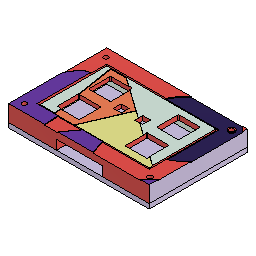
hackpaddelta (Autodesk Fusion 360 design; units mm, degrees)
part number: 2026-03-17-23-30-56-506
Autodesk Fusion 360 part; units mm, degrees
sketch "Sketch3" plane through (0, 0, 0) normal (0, 0, 1) x (1, 0, 0)
  line L0 (0, 0) -> (69.5, 0)
  line L1 (69.5, 0) -> (69.5, 42.5)
  line L2 (69.5, 42.5) -> (0, 42.5)
  line L3 (0, 42.5) -> (0, 0)
  dimension "d5" = 69.5
  dimension "d6" = 42.5
  constraint horizontal L0
  constraint vertical L1
  constraint horizontal L2
  constraint vertical L3
  constraint coincident L0.start L3.end
  measures "d5" distance of L0.start L0.end
  measures "d6" distance of L0.start L2.end
sketch "Sketch11" plane through (0, 0, 0) normal (0, 0, 1) x (1, 0, 0)
  line L0 (0, 0) -> (69.5, 0)
  line L1 (69.5, 0) -> (69.5, 42.5)
  line L2 (69.5, 42.5) -> (0, 42.5)
  line L3 (0, 42.5) -> (0, 0)
  dimension "d46" = 69.5
  dimension "d47" = 42.5
  constraint horizontal L0
  constraint vertical L1
  constraint horizontal L2
  constraint vertical L3
  measures "d46" distance of L0.start L0.end
  measures "d47" distance of L0.start L2.end
sketch "Sketch5" plane through (0, 0, 0) normal (0, 0, 1) x (1, 0, 0)
  line L0 (0, 0) -> (69.5, 0)
  line L1 (69.5, 0) -> (69.5, 42.5)
  line L2 (69.5, 42.5) -> (0, 42.5)
  line L3 (0, 42.5) -> (0, 0)
  line L4 (-10, -10) -> (79.5, -10)
  line L5 (79.5, -10) -> (79.5, 52.5)
  line L6 (79.5, 52.5) -> (-10, 52.5)
  line L7 (-10, 52.5) -> (-10, -10)
  circle A0 centre (-5, 47) radius 1.45
  circle A1 centre (-5, -5) radius 1.45
  circle A2 centre (75, 47) radius 1.45
  circle A3 centre (75, -5) radius 1.45
  dimension "d9" = 69.5
  dimension "d10" = 42.5
  dimension "d11" = 10
  dimension "d12" = 2.9
  dimension "d13" = 2.9
  dimension "d14" = 2.9
  dimension "d15" = 2.9
  constraint horizontal L0
  constraint vertical L1
  constraint horizontal L2
  constraint vertical L3
  constraint coincident L0.start L3.end
  measures "d9" distance of L0.start L0.end
  measures "d10" distance of L0.start L2.end
  measures "d12" diameter of A0
  measures "d13" diameter of A1
  measures "d14" diameter of A2
  measures "d15" diameter of A3
extrude "Extrude1" add sketch "Sketch5" along normal blind 3 contours L0 L1 L2 L3 makes body 1
extrude "Extrude2" add sketch "Sketch5" along normal blind 3 separate body makes body 2
sketch "Sketch6" plane through (0, 0, 3) normal (0, 0, 1) x (-1, 0, 0)
  line L0 (-25.0112, -26.63) -> (-30.0112, -26.63)
  line L1 (-30.0112, -26.63) -> (-30.0112, -21.63)
  line L2 (-30.0112, -21.63) -> (-25.0112, -21.63)
  line L3 (-25.0112, -21.63) -> (-25.0112, -26.63)
  line L4 (-43.6881, -26.63) -> (-38.6881, -26.63)
  line L5 (-38.6881, -26.63) -> (-38.6881, -21.63)
  line L6 (-38.6881, -21.63) -> (-43.6881, -21.63)
  line L7 (-43.6881, -21.63) -> (-43.6881, -26.63)
  dimension "d36" = 5
  dimension "d37" = 5
  dimension "d40" = 5
  dimension "d41" = 5
  constraint horizontal L0
  constraint vertical L1
  constraint horizontal L2
  constraint vertical L3
  constraint horizontal L4
  constraint vertical L5
  constraint horizontal L6
  constraint vertical L7
  measures "d36" distance of L0.start L0.end
  measures "d37" distance of L0.start L2.end
  measures "d40" distance of L4.start L4.end
  measures "d41" distance of L4.start L6.end
extrude "Extrude3" add 1 faces at (73.5198, 14, 3) along direction (0, 0, 1) blind 10 separate body on bodies 2 makes body 3
sketch "Sketch7" plane through (0, 0, 3) normal (0, 0, 1) x (-1, 0, 0)
  arc A0 (-20.375, -18.025) -> (-19.875, -18.525) centre (-19.875, -18.025) ccw
  arc A1 (-6.875, -18.525) -> (-6.375, -18.025) centre (-6.875, -18.025) ccw
  arc A2 (-6.375, -5.025) -> (-6.875, -4.525) centre (-6.875, -5.025) ccw
  arc A3 (-19.875, -4.525) -> (-20.375, -5.025) centre (-19.875, -5.025) ccw
  line L0 (-19.875, -18.525) -> (-6.875, -18.525)
  line L1 (-6.875, -4.525) -> (-19.875, -4.525)
  line L2 (-6.375, -18.025) -> (-6.375, -5.025)
  line L3 (-20.375, -5.025) -> (-20.375, -18.025)
  arc A4 (-6.375, -25.025) -> (-6.875, -24.525) centre (-6.875, -25.025) ccw
  line L4 (-19.875, -38.525) -> (-6.875, -38.525)
  arc A5 (-6.875, -38.525) -> (-6.375, -38.025) centre (-6.875, -38.025) ccw
  arc A6 (-20.375, -38.025) -> (-19.875, -38.525) centre (-19.875, -38.025) ccw
  line L5 (-6.875, -24.525) -> (-19.875, -24.525)
  line L6 (-20.375, -25.025) -> (-20.375, -38.025)
  arc A7 (-19.875, -24.525) -> (-20.375, -25.025) centre (-19.875, -25.025) ccw
  line L7 (-6.375, -38.025) -> (-6.375, -25.025)
  arc A8 (-50.125, -18.525) -> (-49.625, -18.025) centre (-50.125, -18.025) ccw
  line L8 (-50.125, -4.525) -> (-63.125, -4.525)
  arc A9 (-63.125, -4.525) -> (-63.625, -5.025) centre (-63.125, -5.025) ccw
  arc A10 (-49.625, -5.025) -> (-50.125, -4.525) centre (-50.125, -5.025) ccw
  line L9 (-63.625, -5.025) -> (-63.625, -18.025)
  line L10 (-49.625, -18.025) -> (-49.625, -5.025)
  line L11 (-63.125, -18.525) -> (-50.125, -18.525)
  arc A11 (-63.625, -18.025) -> (-63.125, -18.525) centre (-63.125, -18.025) ccw
  arc A12 (-63.625, -38.025) -> (-63.125, -38.525) centre (-63.125, -38.025) ccw
  arc A13 (-63.125, -24.525) -> (-63.625, -25.025) centre (-63.125, -25.025) ccw
  line L12 (-63.625, -25.025) -> (-63.625, -38.025)
  line L13 (-50.125, -24.525) -> (-63.125, -24.525)
  line L14 (-49.625, -38.025) -> (-49.625, -25.025)
  line L15 (-63.125, -38.525) -> (-50.125, -38.525)
  arc A14 (-50.125, -38.525) -> (-49.625, -38.025) centre (-50.125, -38.025) ccw
  arc A15 (-49.625, -25.025) -> (-50.125, -24.525) centre (-50.125, -25.025) ccw
extrude "Extrude4" add 1 faces at (23.1667, 14.1667, 3) along direction (0, 0, -1) blind 3 from surface at -10 on bodies 1 bodies 1 3
extrude "Extrude5" cut sketch "Sketch7" sketch "Sketch6" against normal blind 10 from surface at 10 of sketch 2 bodies 3
sketch "Sketch13" plane through (0, -10, 0) normal (0, -1, 0) x (1, 0, 0)
  line L0 (-10, 3) -> (79.5, 3)
  line L1 (79.5, 3) -> (79.5, 13)
  line L2 (79.5, 13) -> (-10, 13)
  line L3 (-10, 13) -> (-10, 3)
  line L4 (20.5, 9) -> (49.5, 9)
  line L5 (49.5, 9) -> (49.5, 3)
  line L6 (49.5, 3) -> (20.5, 3)
  line L7 (20.5, 3) -> (20.5, 9)
  dimension "d54" = 6
  constraint horizontal L4
  constraint vertical L5
  constraint horizontal L6
  constraint vertical L7
  measures "d54" distance of L4.start L6.end
extrude "Extrude6" cut sketch "Sketch13" against normal blind 10 contours L0 L4 L5 L6 L7 bodies 3
sketch "Sketch14" plane through (0, 0, 13) normal (0, 0, 1) x (-1, 0, 0)
  line L0 (-38.6881, -26.63) -> (-43.6881, -26.63)
  line L1 (-43.6881, -26.63) -> (-43.6881, -21.63)
  line L2 (-43.6881, -21.63) -> (-38.6881, -21.63)
  line L3 (-38.6881, -21.63) -> (-38.6881, -26.63)
  arc A0 (-20.375, -18.025) -> (-19.875, -18.525) centre (-19.875, -18.025) ccw
  line L4 (-20.375, -18.025) -> (-20.375, -5.025)
  arc A1 (-19.875, -4.525) -> (-20.375, -5.025) centre (-19.875, -5.025) ccw
  line L5 (-19.875, -4.525) -> (-6.875, -4.525)
  arc A2 (-6.375, -5.025) -> (-6.875, -4.525) centre (-6.875, -5.025) ccw
  line L6 (-6.375, -5.025) -> (-6.375, -18.025)
  arc A3 (-6.875, -18.525) -> (-6.375, -18.025) centre (-6.875, -18.025) ccw
  line L7 (-6.875, -18.525) -> (-19.875, -18.525)
  line L8 (-50.125, -18.525) -> (-63.125, -18.525)
  arc A4 (-63.625, -18.025) -> (-63.125, -18.525) centre (-63.125, -18.025) ccw
  line L9 (-63.625, -18.025) -> (-63.625, -5.025)
  arc A5 (-63.125, -4.525) -> (-63.625, -5.025) centre (-63.125, -5.025) ccw
  line L10 (-63.125, -4.525) -> (-50.125, -4.525)
  arc A6 (-49.625, -5.025) -> (-50.125, -4.525) centre (-50.125, -5.025) ccw
  line L11 (-49.625, -5.025) -> (-49.625, -18.025)
  arc A7 (-50.125, -18.525) -> (-49.625, -18.025) centre (-50.125, -18.025) ccw
  arc A8 (-6.375, -25.025) -> (-6.875, -24.525) centre (-6.875, -25.025) ccw
  line L12 (-6.375, -25.025) -> (-6.375, -38.025)
  arc A9 (-6.875, -38.525) -> (-6.375, -38.025) centre (-6.875, -38.025) ccw
  line L13 (-6.875, -38.525) -> (-19.875, -38.525)
  arc A10 (-20.375, -38.025) -> (-19.875, -38.525) centre (-19.875, -38.025) ccw
  line L14 (-20.375, -38.025) -> (-20.375, -25.025)
  arc A11 (-19.875, -24.525) -> (-20.375, -25.025) centre (-19.875, -25.025) ccw
  line L15 (-19.875, -24.525) -> (-6.875, -24.525)
  line L16 (-63.125, -24.525) -> (-50.125, -24.525)
  arc A12 (-49.625, -25.025) -> (-50.125, -24.525) centre (-50.125, -25.025) ccw
  line L17 (-49.625, -25.025) -> (-49.625, -38.025)
  arc A13 (-50.125, -38.525) -> (-49.625, -38.025) centre (-50.125, -38.025) ccw
  line L18 (-50.125, -38.525) -> (-63.125, -38.525)
  arc A14 (-63.625, -38.025) -> (-63.125, -38.525) centre (-63.125, -38.025) ccw
  line L19 (-63.625, -38.025) -> (-63.625, -25.025)
  arc A15 (-63.125, -24.525) -> (-63.625, -25.025) centre (-63.125, -25.025) ccw
  line L20 (-30.0112, -26.63) -> (-30.0112, -21.63)
  line L21 (-30.0112, -21.63) -> (-25.0112, -21.63)
  line L22 (-25.0112, -21.63) -> (-25.0112, -26.63)
  line L23 (-25.0112, -26.63) -> (-30.0112, -26.63)
  circle A16 centre (5, 5) radius 1.45
  circle A17 centre (5, -47) radius 1.45
  circle A18 centre (-75, 5) radius 1.45
  circle A19 centre (-75, -47) radius 1.45
  line L24 (10, -52.5) -> (10, 10)
  line L25 (10, 10) -> (-79.5, 10)
  line L26 (-79.5, 10) -> (-79.5, -52.5)
  line L27 (-79.5, -52.5) -> (10, -52.5)
  line L28 (-69.5, -42.5) -> (0, -42.5)
  line L29 (0, -42.5) -> (0, 0)
  line L30 (0, 0) -> (-69.5, 0)
  line L31 (-69.5, 0) -> (-69.5, -42.5)
  line L32 (-70.5, -43.5) -> (1, -43.5)
  line L33 (1, -43.5) -> (1, 1)
  line L34 (1, 1) -> (-70.5, 1)
  line L35 (-70.5, 1) -> (-70.5, -43.5)
  circle A20 centre (-75, -47) radius 2.05
  dimension "d57" = 1
  dimension "d64" = 4.1
  constraint horizontal L28
  constraint vertical L29
  constraint horizontal L30
  constraint vertical L31
  constraint concentric A19 A20
  measures "d64" diameter of A20
extrude "Extrude7" cut sketch "Sketch14" against normal blind 1 contours L32 L33 L34 L35 bodies 3
sketch "Sketch15" plane through (0, 0, 13) normal (0, 0, 1) x (-1, 0, 0)
  line L0 (10, -52.5) -> (10, 10)
  line L1 (10, 10) -> (-79.5, 10)
  line L2 (-79.5, 10) -> (-79.5, -52.5)
  line L3 (-79.5, -52.5) -> (10, -52.5)
  circle A0 centre (-75, -47) radius 1.45
  circle A1 centre (-75, 5) radius 1.45
  circle A2 centre (5, -47) radius 1.45
  circle A3 centre (5, 5) radius 1.45
  line L4 (1, -43.5) -> (-70.5, -43.5)
  line L5 (-70.5, -43.5) -> (-70.5, 1)
  line L6 (-70.5, 1) -> (1, 1)
  line L7 (1, 1) -> (1, -43.5)
  circle A4 centre (-60, -33) radius 25.4558
form "Form1" [no effect]
emboss "Emboss1" depth -0.5 profiles "Sketch15" section 1 contours L2 L3 L4 L5 A4 onto face at (73.8532, 13.6667, 13) on bodies 3 bodies 3
extrude "Extrude8" add sketch "Sketch14" along normal blind 0.5 from surface at -0.5 contours A20 bodies 3
sketch "Sketch16" plane through (0, 0, 13) normal (0, 0, 1) x (-1, 0, 0)
  line L0 (0, 0) -> (-69.5, 0)
  line L1 (-69.5, 0) -> (-69.5, -42.5)
  line L2 (-69.5, -42.5) -> (0, -42.5)
  line L3 (0, -42.5) -> (0, 0)
  line L4 (-12.3802, -42.5) -> (-69.5, -2.1183)
  line L5 (-33.7676, -27.3799) -> (-22, 0)
  line L6 (-2.5619, -42.5) -> (-11, 10)
  constraint horizontal L0
  constraint vertical L1
  constraint horizontal L2
  constraint vertical L3
  constraint coincident L0.start L3.end
  constraint coincident L2 L4.start
  constraint coincident L1 L4.end
  constraint coincident L4 L5.start
  constraint coincident L0 L5.end
  constraint coincident L2 L6.start
extrude "Extrude10" cut sketch "Sketch16" against normal blind 0.5 contours L0 L2 L4 L5 L6 bodies 3
extrude "Extrude11" cut sketch "Sketch16" against normal blind 0.25 contours L0 L1 L4 L5 bodies 3
sketch "Sketch19" plane through (0, 0, 13) normal (0, 0, 1) x (-1, 0, 0)
  circle A0 centre (5, 5) radius 1.45
  circle A1 centre (5, -47) radius 1.45
  circle A2 centre (-75, 5) radius 1.45
  arc A3 (-43.6369, -52.5) -> (-36.8106, -43.5) centre (-60, -33) ccw
  line L0 (-43.6369, -52.5) -> (10, -52.5)
  line L1 (10, -52.5) -> (10, 10)
  line L2 (10, 10) -> (-79.5, 10)
  line L3 (-79.5, 10) -> (-79.5, -16.6369)
  arc A4 (-70.5, -9.8106) -> (-79.5, -16.6369) centre (-60, -33) ccw
  line L4 (-70.5, -9.8106) -> (-70.5, 1)
  line L5 (-70.5, 1) -> (1, 1)
  line L6 (1, 1) -> (1, -43.5)
  line L7 (1, -43.5) -> (-36.8106, -43.5)
  spline S0 degree 5 poles (10, -24) (9.4395, -25.1505) (8.3108, -27.2732) (6.5951, -29.9228) (4.262, -32.3847) (1.2869, -33.6716) (-1.6958, -33.1718) (-4.5794, -30.9066) (-7.1965, -26.9306) (-9.3745, -21.381) (-10.9804, -14.5194) (-11.9734, -6.783) (-12.4473, 1.179) (-12.6977, 8.428) (-13.1411, 13.9208) (-14.1926, 16.7728) (-16.163, 16.483) (-19.1352, 13.2084) (-22.8836, 7.9295) (-27.0121, 2.0619) (-31.0617, -2.8572) (-34.6319, -5.5148) (-37.4906, -5.1417) (-39.7036, -1.8849) (-41.5551, 3.4343) (-43.4485, 9.623) (-45.8203, 15.3774) (-49.0358, 19.5996) (-53.3393, 21.5509) (-58.8888, 20.7479) (-65.7712, 16.9201) (-72.3739, 11.3396) (-77.9462, 5.7247) (-81.9362, 1.3473) (-84, -1) knots 0 0 0 0 0 0 0.033333 0.066667 0.1 0.133333 0.166667 0.2 0.233333 0.266667 0.3 0.333333 0.366667 0.4 0.433333 0.466667 0.5 0.533333 0.566667 0.6 0.633333 0.666667 0.7 0.733333 0.766667 0.8 0.833333 0.866667 0.9 0.933333 0.966667 1 1 1 1 1 1
  point P0 (-1, -33)
  point P1 (-12, -5)
  point P2 (-16, 16)
  point P3 (-34.75, -4.8555)
  point P4 (-45, 13)
  constraint coincident L1 S0.start
extrude "Extrude12" add sketch "Sketch19" along normal blind 0.5 separate body contours L2 L5 S0 picked at (-31.0465, 7) makes body 4
extrude "Extrude13" add sketch "Sketch19" along normal blind 0.5 separate body contours L1 L2 L5 L6 S0 makes body 5
extrude "Extrude14" add sketch "Sketch19" along normal blind 0.5 separate body contours L2 L3 S0 makes body 6
combine "Combine1" operation add target body 1 tool bodies 2
combine "Combine2" operation add target body 3 tool bodies 4 5 6
